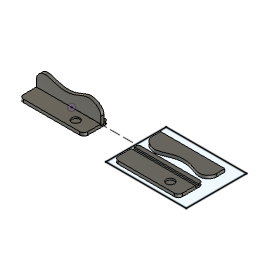
2025-Basic-CNC-Project (Autodesk Fusion 360 design; units mm, degrees)
Autodesk Fusion 360 part; units mm, degrees
sketch "Sketch1" plane through (0, 0, 0) normal (0, 0, 1) x (1, 0, 0) in component "Base"
  line L0 (-200, 25) -> (200, 25)
  line L1 (200, 25) -> (200, -125)
  line L2 (200, -125) -> (-200, -125)
  line L3 (-200, -125) -> (-200, 25)
  line L4 (-200, 25) -> (0, 0) construction
  line L5 (0, 0) -> (200, 25) construction
  dimension "d1" = 150
  dimension "d2" = 400
  dimension "d3" = 25
  constraint horizontal L0
  constraint vertical L1
  constraint horizontal L2
  constraint vertical L3
  constraint coincident L4.end L5.start
  constraint coincident L0 L1.start
  constraint equal L4 L5
  constraint coincident L0.end L1.start
  measures "d1" distance of L0.start L2.end
  measures "d2" distance of L0.start L0.end
  measures "d3" distance of L4.end L0
extrude "Extrude1" add sketch "Sketch1" along normal blind 19 makes body 1 in component "Base"
fillet "Fillet1" radius 25 2 edges at (-200, -125, 9.5) (200, -125, 9.5) on bodies 1 in component "Base"
fillet "Fillet2" radius 15 2 edges at (200, 25, 9.5) (-200, 25, 9.5) on bodies 1 in component "Base"
sketch "Sketch1 (2)" plane through (0, 0, 0) normal (0, 1, 0) x (1, 0, 0) in component "Back Piece"
  line L0 (-200, -9.5) -> (-200, -59.5)
  line L1 (200, -9.5) -> (200, -59.5)
  line L2 (200, -59.5) -> (200, -9.5)
  line L3 (-200, -9.5) -> (200, -9.5)
  spline S0 degree 5 poles (-200, -59.5) (-200, -62.5478) (-200, -68.6434) (-198.1266, -79.4984) (-187.9451, -97.9965) (-163.0177, -116.2577) (-131.7996, -115.191) (-97.0355, -101.2384) (-59.1553, -89.1058) (-20.3737, -83.9005) (17.5796, -88.56) (53.3559, -101.2392) (86.6815, -117.0645) (119.2533, -127.3246) (154.7132, -120.5252) (184.7241, -101.2489) (197.6261, -82.7944) (200, -70.6956) (200, -63.2319) (200, -59.5) knots 0 0 0 0 0 0 0.066667 0.133333 0.2 0.266667 0.333333 0.4 0.466667 0.533333 0.6 0.666667 0.733333 0.8 0.866667 0.933333 1 1 1 1 1 1
  line L4 (51.7037, -107.059) -> (148.2963, -132.941)
  line L5 (-182.5737, -121.1824) -> (-84.0929, -103.8176)
  line L6 (-200, -39.5) -> (-200, -79.5)
  line L7 (200, -79.5) -> (200, -39.5)
  line L8 (-175, -19) -> (-200, -19) construction
  line L9 (-175, -19) -> (175, -19) construction
  line L10 (200, -19) -> (175, -19) construction
  line L11 (200, 0) -> (200, -19) construction
  line L12 (175, 0) -> (200, 0)
  line L13 (175, 0) -> (-175, 0) construction
  line L14 (-200, -19) -> (-200, 0) construction
  line L15 (-200, 0) -> (-175, 0) construction
  point P0 (-133.3333, -112.5)
  point P1 (100, -120)
  dimension "d11" = 50
  dimension "d12" = 40
  dimension "d13" = 40
  dimension "d14" = 100
  dimension "d15" = 10
  dimension "d16" = 15
  dimension "d20" = 120
  dimension "d32" = 133.3333
  dimension "d33" = 112.5
  dimension "d34" = 100
  dimension "d35" = 9.5
  constraint horizontal L3
  constraint perpendicular L0 L3
  constraint perpendicular L2 L3
  constraint horizontal L0.end L1.end
  constraint coincident L1.end L2.start
  constraint midpoint P1 L4
  constraint midpoint P0 L5
  constraint midpoint L0.end L6
  constraint midpoint L1.end L7
  constraint equal L4 L5
  constraint coincident L0.start L14
  constraint coincident L1.start L11
  measures "d11" distance of L1.start L1.end
  measures "d12" distance of L7.start L7.end
  measures "d13" distance of L6.start L6.end
  measures "d14" distance of L5.start L5.end
  measures "d15" angle of L3 L5
  measures "d16" angle of L3 L4
  measures "d20" vertical distance of origin P1
  measures "d32" horizontal distance of origin P0
  measures "d33" vertical distance of origin P0
  measures "d34" horizontal distance of origin P1
  measures "d35" distance of L3 L9
extrude "Extrude1'" add sketch "Sketch1 (2)" against normal blind 19 separate body makes body 2 in component "Back Piece"
combine "Combine1" operation cut target body 1 tool bodies 2 keep tools in component "Base"
sketch "Sketch1 (3)" plane through (0, 0, 19) normal (0, 0, 1) x (-1, 0, 0) in component "Base"
  line L0 (-200, 19) -> (200, 19)
  arc A0 (200, 100) -> (175, 125) centre (175, 100) ccw
  line L1 (175, 125) -> (-175, 125)
  arc A1 (-175, 125) -> (-200, 100) centre (-175, 100) ccw
  circle A2 centre (-100, 75) radius 25
  line L2 (200, 19) -> (200, 100)
  line L3 (-200, 100) -> (-200, 19)
  dimension "d27" = 50
  dimension "d28" = 100
  dimension "d29" = 75
  measures "d27" diameter of A2
  measures "d28" horizontal distance of origin A2.centre
  measures "d29" vertical distance of origin A2.centre
extrude "Extrude2" cut sketch "Sketch1 (3)" against normal blind 9.5 contours A2 bodies 1 in component "Base"
sketch "plywood" plane through (0, 0, 0) normal (0, 0, 1) x (1, 0, 0)
  line L0 (400, 187.5) -> (900, 187.5)
  line L1 (900, 187.5) -> (900, -187.5)
  line L2 (900, -187.5) -> (400, -187.5)
  line L3 (400, -187.5) -> (400, 187.5)
  line L4 (0, 0) -> (400, 0) construction
  dimension "d36" = 500
  dimension "d37" = 375
  dimension "d38" = 400
  constraint horizontal L0
  constraint vertical L1
  constraint horizontal L2
  constraint vertical L3
  constraint coincident L4.start origin
  constraint coincident L3 L4.end
  constraint perpendicular L3 L4
  constraint midpoint L3 L4.end
  measures "d36" distance of L0.start L0.end
  measures "d37" distance of L0.start L2.end
  measures "d38" distance of L4.start L4.end
other "Arrange1"
component "Base" placed x (1, 0, 0) y (0, 1, 0) z (0, 0, 1) at (0, 0, 0)
component "Back Piece" placed x (1, 0, 0) y (0, 1, 0) z (0, 0, 1) at (0, 0, 0)
component "Arrange1" placed x (1, 0, 0) y (0, 1, 0) z (0, 0, 1) at (0, 0, 0)
component "Envelope1(Qty: 1)" placed x (1, 0, 0) y (0, 1, 0) z (0, 0, 1) at (400, -187.5, 0) in component "Arrange1"
component "Base" placed x (1, 0, 0) y (0, 1, 0) z (0, 0, 1) at (225.4, 150.4, 0) in component "Envelope1(Qty: 1)"
component "Back Piece" placed x (-1, 0, 0) y (0, 0, -1) z (0, -1, 0) at (225.4015, 323.9804, 0) in component "Envelope1(Qty: 1)"
equation "d1 = depth"
equation "d2 = width"
equation "d3 = depth / 6"
equation "width = 400 mm"
equation "depth = width * 0.375"
equation "ply = 19 mm"
equation "d8 = ply"
equation "d11 = depth / 3"
equation "d12 = width / 10"
equation "d13 = width / 10"
equation "d14 = width / 4"
equation "d20 = depth * 0.8"
equation "d21 = -ply"
equation "d24 = width / 16"
equation "d26 = depth * 0.1"
equation "d27 = depth / 3"
equation "d28 = width / 4"
equation "d29 = depth / 2"
equation "d30 = -ply / 2"
equation "d32 = width / 3"
equation "d33 = depth * 0.75"
equation "d34 = width / 4"
equation "d35 = ply / 2"
equation "d36 = width * 1.25"
equation "d37 = depth * 2.5"
equation "d38 = width"
